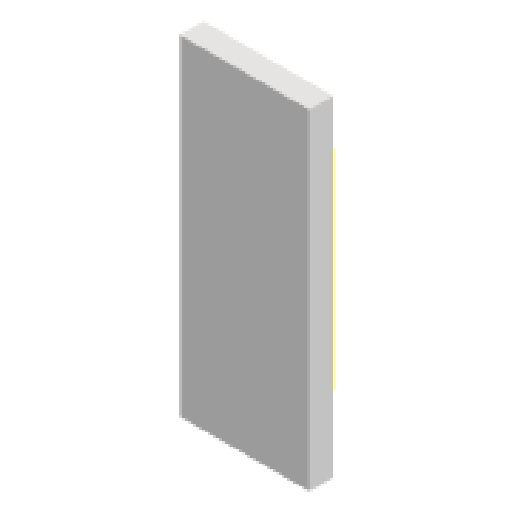
# Autodesk Inventor part: Рейка
Saved by Autodesk Inventor 2026 (Build 300175000, 175)
## iProperties
Created: 2026-04-20
Part Number: Рейка
Material: Типовые
Document SubType Name: Modeling
Designer: Artem Sannikov
Density: 1 g/cm^3
Appearance: По умолчанию
Author: Artem Sannikov
Autodesk Inventor part; units mm, degrees
ref_plane "YZ Plane" through (0, 0, 0) normal (1, 0, 0) x (0, 1, 0)
ref_plane "XZ Plane" through (0, 0, 0) normal (0, 1, 0) x (-1, 0, 0)
ref_plane "XY Plane" through (0, 0, 0) normal (0, 0, 1) x (1, 0, 0)
ref_plane "РабПлоскость1" through (0, 0, 0) normal (0, 0, 1) x (1, 0, 0)
sketch "Эскиз1" plane through (0, 0, 0) normal (0, 0, 1) x (1, 0, 0)
  line L0 (26.2263, -17.9063) -> (-1.0249, -17.9063)
  line L1 (-1.0249, -17.9063) -> (-1.0249, 51.5483)
  line L2 (-1.0249, 51.5483) -> (26.2263, 51.5483)
  line L3 (26.2263, 51.5483) -> (26.2263, -17.9063)
  line L4 (26.2263, -17.9063) -> (-1.0249, 51.5483) construction
  line L5 (-1.0249, -17.9063) -> (26.2263, 51.5483) construction
  point P0 (0, 0)
  point P1 (12.6007, 16.821)
  constraints: 12 end point, 2 midpoint, 2 parallel, 1 horizontal, 1 perpendicular
extrude "Выдавливание1" add sketch "Эскиз1" along normal blind 5
